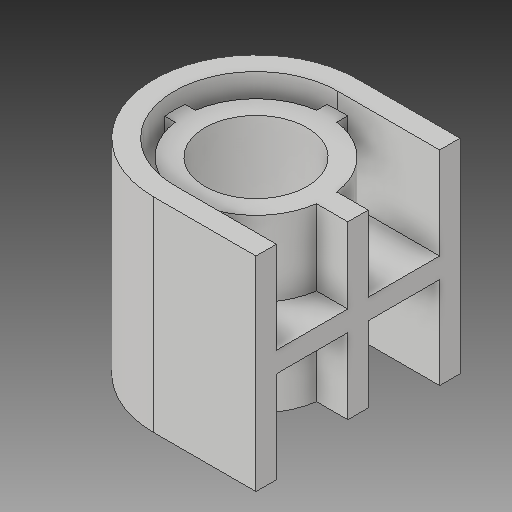
# Autodesk Inventor part: straight_beam_end_part_single
Saved by Autodesk Inventor 2019 (Build 230136000, 136)
## iProperties
Created: 2019-01-31
Part Number: straight_beam_end_part_single
Material: Generic
Document SubType Name: Modeling
Designer: Varga Daniel
Density: 1 g/cm^3
Appearance: Default
Author: Varga Daniel
Autodesk Inventor part; units mm, degrees
ref_plane "YZ Plane" through (0, 0, 0) normal (1, 0, 0) x (0, 1, 0)
ref_plane "XZ Plane" through (0, 0, 0) normal (0, 1, 0) x (-1, 0, 0)
derived "Base_part.ipt"
sketch "Sketch1" plane through (0, 0, 0) normal (0, 1, 0) x (-1, 0, 0)
  line L0 (5, 0) -> (25, 0)
  line L1 (30, 5) -> (30, 25)
  line L2 (25, 30) -> (5, 30)
  line L3 (0, 25) -> (0, 5)
  line L4 (5, 29) -> (25, 29)
  line L5 (29, 25) -> (29, 5)
  line L6 (25, 1) -> (5, 1)
  line L7 (1, 5) -> (1, 25)
  circle A0 centre (5, 5) radius 2.5
  circle A1 centre (5, 5) radius 3.5
  arc A2 (25, 0) -> (30, 5) centre (25, 5) ccw
  arc A3 (30, 25) -> (25, 30) centre (25, 25) ccw
  arc A4 (5, 30) -> (0, 25) centre (5, 25) ccw
  arc A5 (0, 5) -> (5, 0) centre (5, 5) ccw
  arc A6 (1, 5) -> (5, 1) centre (5, 5) ccw
  arc A7 (5, 29) -> (1, 25) centre (5, 25) ccw
  arc A8 (29, 25) -> (25, 29) centre (25, 25) ccw
  arc A9 (25, 1) -> (29, 5) centre (25, 5) ccw
  line L8 (49.1041, 15) -> (-27.081, 15) construction
  line L9 (31.1478, 10) -> (-2.4877, 10) construction
  line L10 (-2.8604, 5) -> (35.495, 5) construction
  line L11 (5, -2.5736) -> (5, 36.7522) construction
  line L12 (15, -1.4978) -> (15, 34.8784) construction
  line L13 (1.5359, 5.5) -> (1, 5.5)
  line L14 (1.5359, 4.5) -> (1.0314, 4.5)
  line L15 (28.9686, 4.5) -> (8.4641, 4.5)
  line L16 (29, 5.5) -> (8.4641, 5.5)
  line L17 (4.5, 1.5359) -> (4.5, 1.0314)
  line L18 (5.5, 1.5359) -> (5.5, 1)
  line L19 (29, 10.5) -> (1, 10.5)
  line L20 (29, 9.5) -> (1, 9.5)
  line L21 (4.5, 28.9686) -> (4.5, 10.5)
  line L22 (4.5, 9.5) -> (4.5, 8.4641)
  line L23 (5.5, 29) -> (5.5, 10.5)
  line L24 (5.5, 9.5) -> (5.5, 8.4641)
  point P0 (0, 0)
  point P1 (30, 30)
  point P2 (0, 30)
  point P3 (5, 25)
sketch "Sketch3" plane through (0, 0, 0) normal (0, 1, 0) x (-1, 0, 0)
  circle A0 centre (5, 5) radius 2.5 construction
  circle A1 centre (5, 5) radius 3.5 construction
  circle A2 centre (5, 5) radius 2.5
  arc A3 (4.5, 1.5359) -> (1.5359, 5.5) centre (5, 5) ccw
  line L0 (0.3508, 5) -> (13.598, 5) construction
  line L1 (5, 13.9543) -> (5, -1.7484) construction
  line L2 (5, 10) -> (0, 10)
  line L3 (0, 10) -> (0, 9)
  line L4 (0, 9) -> (2, 9)
  line L5 (0, 1) -> (0, 0)
  line L6 (0, 0) -> (5, 0)
  line L7 (0, 0) -> (0, 1)
  line L8 (1.5359, 5.5) -> (0, 5.5)
  line L9 (0, 5.5) -> (0, 4.5)
  line L10 (0, 4.5) -> (1.5359, 4.5)
  line L11 (0, 9) -> (4.5, 9)
  line L12 (0, 9) -> (0, 10)
  line L13 (5, 9) -> (5, 9)
  arc A4 (5, 0) -> (5, 10) centre (5, 5) ccw
  line L14 (5, 1) -> (4.5, 1)
  arc A5 (5, 1) -> (8.9686, 4.5) centre (5, 5) ccw
  line L15 (4.5, 9) -> (4.5, 8.4641)
  line L16 (5.5, 8.9686) -> (5.5, 8.4641)
  line L17 (5.5, 1.0314) -> (5.5, 1.5359)
  line L18 (4.5, 1.5359) -> (4.5, 1)
  line L19 (8.4641, 5.5) -> (8.9686, 5.5)
  line L20 (8.4641, 4.5) -> (8.9686, 4.5)
  line L21 (0, 1) -> (0, 4.5)
  line L22 (0, 4.5) -> (0, 5.5)
  line L23 (0, 5.5) -> (0, 9)
  line L24 (4.5, 9) -> (5, 9)
  arc A6 (8.9686, 5.5) -> (5, 9) centre (5, 5) ccw
  arc A7 (8.9686, 4.5) -> (8.9686, 5.5) centre (5, 5) ccw
  arc A8 (1.5359, 4.5) -> (4.5, 1.5359) centre (5, 5) ccw
  arc A9 (1.5359, 5.5) -> (1.5359, 4.5) centre (5, 5) ccw
  line L25 (4.5, 1) -> (0, 1)
  line L26 (2, 9) -> (4.5, 9)
  line L27 (4.5, 9) -> (5, 9)
  point P0 (0, 0)
  dimension "d2" = 10
  dimension "d5" = 1
  dimension "d20" = 1
  dimension "d21" = 5
  dimension "d22" = 1
  dimension "d23" = 1
  constraints: 56 end point, 31 point on circle, 14 perpendicular, 10 parallel, 9 point on line, 8 centre point, 7 tangent, 5 collinear, 4 horizontal, 2 coincident, 2 concentric, 1 vertical, 3 other
  measures "d2" distance between parallel lines of L2 L6
  measures "d5" distance between parallel lines of L2 L4
  measures "d20" distance between parallel lines of L8 L10
  measures "d21" distance between parallel lines of L1 L7
  measures "d22" distance between parallel lines of L6 L14
  measures "d23" distance between parallel lines of L15 L16
ref_plane "Work Plane2" through (0, 0, 5.5) normal (0, 1, 0) x (0, 0, 1)
extrude "Extrusion7" add sketch "Sketch3" along normal blind 5 contours L14 A5 A7 A6 L24 L11 L4 L3 L2 A4 L6 L5 L25
extrude "Extrusion8" add sketch "Sketch3" against normal blind 5 contours L14 A5 A7 A6 L24 L11 L4 L3 L2 A4 L6 L5 L25
extrude "Extrusion9" add sketch "Sketch3" along normal blind 4.2 contours A8 A9 A3 | A3 L17 A5 L14 L18 | L10 L9 L8 A9 | A3 L19 A7 L20 | L15 L24 A6 L16 A3
extrude "Extrusion10" add sketch "Sketch3" against normal blind 4.2 contours A8 A9 A3 | A3 L17 A5 L14 L18 | L10 L9 L8 A9 | A3 L19 A7 L20 | L15 L24 A6 L16 A3
extrude "Extrusion13" add sketch "Sketch3" along normal blind 0.5 contours L18 L25 L21 L10 A8 | A3 L20 A5 L17 | L8 L23 L4 L11 L15 A3 | A3 L16 A6 L19
extrude "Extrusion14" add sketch "Sketch3" against normal blind 0.5 contours L18 L25 L21 L10 A8 | A3 L20 A5 L17 | L8 L23 L4 L11 L15 A3 | A3 L16 A6 L19
equation "\"d5\" = Wall_thickness"
equation "\"d20\" = Inner_route_thickness"
equation "\"d23\" = Inner_route_thickness"
equation "\"d24\" = 0.5 * Overall_height"
equation "\"d26\" = 0.5 * Overall_height"
equation "\"d28\" = 0.5 * Hole_height"
equation "\"d30\" = 0.5 * Hole_height"
equation "\"d36\" = 0.5 * Inner_thickness"
equation "\"d38\" = 0.5 * Inner_thickness"
equation "\"d4\" = Wall_thickness"
equation "\"d7\" = Inner_route_thickness"
equation "\"Wall_thickness\" = 1"
equation "\"Inner_route_thickness\" = 1"
equation "\"Overall_height\" = 10"
equation "\"Hole_height\" = 8.4"
equation "\"Inner_thickness\" = 1"
body "Solid2"
